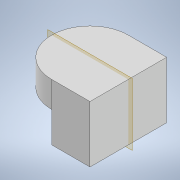
# Autodesk Inventor part: Bending Tool
Saved by Autodesk Inventor 2022.2 (Build 262287000, 287)
## iProperties
Created: 2022-08-14
Part Number: Bending Tool
Material: Generic
Document SubType Name: Modeling
Designer: Ilewicz
Density: 1 g/cm^3
Appearance: Default
Author: Ilewicz
Autodesk Inventor part; units mm, degrees
ref_plane "YZ Plane" through (0, 0, 0) normal (1, 0, 0) x (0, 1, 0)
ref_plane "XZ Plane" through (0, 0, 0) normal (0, 1, 0) x (-1, 0, 0)
ref_plane "XY Plane" through (0, 0, 0) normal (0, 0, 1) x (1, 0, 0)
derived "Crank.ipt"
sketch "Sketch1" plane through (0, 0, 0) normal (0, 1, 0) x (-1, 0, 0)
  arc A0 (0, -2.5) -> (0, 2.5) centre (0, 0) ccw
  line L0 (0, 2.5) -> (-2.5, 2.5)
  line L1 (-2.5, 2.5) -> (-2.5, -2.5)
  line L2 (-2.5, -2.5) -> (0, -2.5)
  dimension "d1" = 2.5
  dimension "d2" = 2.5
  dimension "d3" = 5
  constraints: 6 end point, 2 perpendicular, 2 point on circle, 1 centre point, 1 coincident, 1 horizontal
  measures "d1" radius of A0
  measures "d2" distance of L0.start L0.end
  measures "d3" distance of L0.end L1.end
extrude "Extrusion1" add sketch "Sketch1" along normal blind 3.7
ref_plane "Work Plane2" through (0, 0, 0) normal (0, 0, 1) x (1, 0, 0)
sketch "Sketch3" plane through (0, 0, 0) normal (0, 0, 1) x (1, 0, 0)
  line L0 (-2.5, 0) -> (-2.5, 3.7) projected
  line L1 (-2.5, 0) -> (-2.5, 2)
  line L2 (-2.5, 2) -> (-0.5, 0)
  line L3 (-0.5, 0) -> (-2.5, 0)
  line L4 (0, -0.5) -> (0, 5.2973) construction
  point P0 (0, 0)
  dimension "d9" = 2
  dimension "d10" = 45
  constraints: 8 end point, 2 point on line, 1 perpendicular, 1 vertical
  measures "d9" distance of L1.start L1.end
  measures "d10" angle of L1 L2
revolve "Revolution1" cut sketch "Sketch3" angle 180 mid plane about axis through (0, -0.5, 0) along (0, 1, 0)
equation "\"d1\" = r_tool"
equation "\"d2\" = r_tool"
equation "\"d3\" = 2 * r_tool"
equation "\"r_tool\" = 2.5"
body "Solid1"
